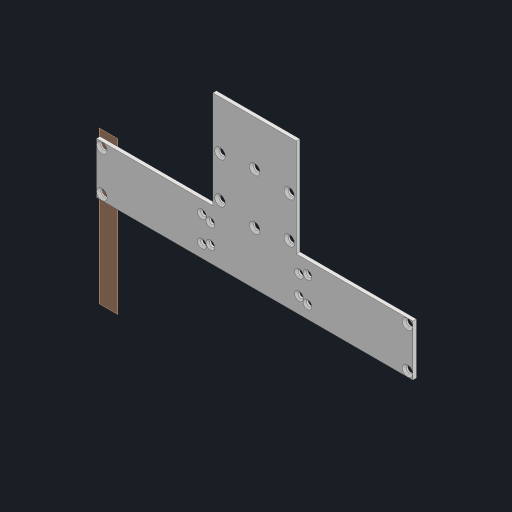
# Autodesk Inventor part: ceil
Saved by Autodesk Inventor 2023 (Build 270158000, 158)
## iProperties
Created: 2024-04-25
Part Number: ceil
Material: Generic
Document SubType Name: Modeling
Designer: szymo
Density: 1 g/cm^3
Appearance: Default
Author: szymo
Autodesk Inventor part; units mm, degrees
ref_plane "YZ Plane" through (0, 0, 0) normal (1, 0, 0) x (0, 1, 0)
ref_plane "XZ Plane" through (0, 0, 0) normal (0, 1, 0) x (-1, 0, 0)
ref_plane "XY Plane" through (0, 0, 0) normal (0, 0, 1) x (1, 0, 0)
ref_plane "Work Plane1" through (0, 0, 0) normal (0, 0, 1) x (1, 0, 0)
ref_plane "Work Plane2" through (0, 0, 0) normal (0, 0, 1) x (1, 0, 0)
sketch "Sketch3" plane through (0, 0, 0) normal (0, 0, 1) x (1, 0, 0)
  circle A0 centre (3, -25.75) radius 2.3 projected
  circle A1 centre (3, -3) radius 2.3 projected
  circle A2 centre (3, -74.8889) radius 2.3 projected
  line L0 (0, 0) -> (6, 0) projected
  line L1 (0, -77.8889) -> (0, 0) projected
  line L2 (0, -77.8889) -> (6, -77.8889) projected
  line L3 (6, -71.8889) -> (6, -77.8889) projected
  line L4 (6, -71.8889) -> (1.6, -71.8889) projected
  line L5 (1.6, -71.8889) -> (1.6, -56.7889) projected
  line L6 (1.6, -56.7889) -> (9.6, -56.7889) projected
  line L7 (9.6, -44.7889) -> (9.6, -56.7889) projected
  line L8 (3, -44.7889) -> (9.6, -44.7889) projected
  line L9 (3, -28.75) -> (3, -44.7889) projected
  line L10 (3, -28.75) -> (6, -28.75) projected
  line L11 (6, -28.75) -> (6, -22.75) projected
  line L12 (6, -22.75) -> (3, -22.75) projected
  line L13 (3, -6) -> (3, -22.75) projected
  line L14 (3, -6) -> (6, -6) projected
  line L15 (6, -6) -> (6, 0) projected
  circle A3 centre (5.6, -52.7889) radius 2.6 projected
  circle A4 centre (175, -3) radius 2.3 projected
  circle A5 centre (175, -25.75) radius 2.3 projected
  line L16 (175, -28.75) -> (175, -41.8889) projected
  line L17 (168.4, -41.8889) -> (175, -41.8889) projected
  line L18 (168.4, -53.8889) -> (168.4, -41.8889) projected
  line L19 (175, -53.8889) -> (168.4, -53.8889) projected
  line L20 (175, -53.8889) -> (175, -71.8889) projected
  line L21 (175, -71.8889) -> (172, -71.8889) projected
  line L22 (172, -71.8889) -> (172, -77.8889) projected
  line L23 (178, -77.8889) -> (172, -77.8889) projected
  line L24 (178, -77.8889) -> (178, 0) projected
  line L25 (178, 0) -> (172, 0) projected
  line L26 (172, 0) -> (172, -6) projected
  line L27 (172, -6) -> (175, -6) projected
  line L28 (175, -6) -> (175, -22.75) projected
  line L29 (175, -22.75) -> (172, -22.75) projected
  line L30 (172, -22.75) -> (172, -28.75) projected
  line L31 (172, -28.75) -> (175, -28.75) projected
  circle A6 centre (175, -74.8889) radius 2.3 projected
  circle A7 centre (172.4, -49.8889) radius 2.6 projected
  circle A8 centre (89, 0.9661) radius 2.3 projected
  circle A9 centre (89, 29.5) radius 2.3 projected
  circle A10 centre (89, 15.55) radius 3.3 projected
  circle A11 centre (89, -14.375) radius 3.3 projected
  circle A12 centre (89, 41.2) radius 3.3 projected
  line L32 (93.5, -27.75) -> (84.5, -27.75) projected
  line L33 (93.5, 55) -> (93.5, -27.75) projected
  line L34 (84.5, 55) -> (93.5, 55) projected
  line L35 (84.5, -27.75) -> (84.5, 55) projected
  line L36 (105.5, -27.75) -> (111.5, -27.75) projected
  line L37 (111.5, -24.9105) -> (111.5, -27.75) projected
  arc A13 (105.5, -24.9105) -> (111.5, -24.9105) centre (108.5, -23.95) ccw projected
  line L38 (105.5, -27.75) -> (105.5, -24.9105) projected
  arc A14 (111.5, -22.9895) -> (105.5, -22.9895) centre (108.5, -23.95) ccw projected
  line L39 (111.5, -5.5855) -> (111.5, -22.9895) projected
  arc A15 (105.5, -5.5855) -> (111.5, -5.5855) centre (108.5, -4.625) ccw projected
  line L40 (105.5, -22.9895) -> (105.5, -5.5855) projected
  circle A16 centre (108.4846, 4.5875) radius 2.3 projected
  arc A17 (105.5, 12.8395) -> (111.5, 12.8395) centre (108.5, 13.8) ccw projected
  line L41 (105.5, -3.6645) -> (105.5, 12.8395) projected
  arc A18 (111.5, -3.6645) -> (105.5, -3.6645) centre (108.5, -4.625) ccw projected
  line L42 (111.5, 12.8395) -> (111.5, -3.6645) projected
  circle A19 centre (108.4462, 27.5) radius 2.3 projected
  arc A20 (111.5, 14.7605) -> (105.5, 14.7605) centre (108.5, 13.8) ccw projected
  line L43 (111.5, 40.6331) -> (111.5, 14.7605) projected
  arc A21 (105.5, 40.1338) -> (111.5, 40.6331) centre (108.4231, 41.3077) ccw projected
  line L44 (105.5, 14.7605) -> (105.5, 40.1338) projected
  arc A22 (111.5, 41.9823) -> (105.5, 42.4816) centre (108.4231, 41.3077) ccw projected
  line L45 (111.5, 55) -> (111.5, 41.9823) projected
  line L46 (105.5, 55) -> (111.5, 55) projected
  line L47 (105.5, 42.4816) -> (105.5, 55) projected
  line L48 (111.5, 41.9823) -> (111.5, 55) projected
  line L49 (111.5, 41.9823) -> (112.5, 41.9823) projected
  line L50 (112.5, 41.9823) -> (112.5, 55) projected
  line L51 (111.5, 55) -> (112.5, 55) projected
  line L52 (111.5, 14.7605) -> (111.5, 40.6331) projected
  line L53 (111.5, 14.7605) -> (112.5, 14.7605) projected
  line L54 (112.5, 14.7605) -> (112.5, 40.6331) projected
  line L55 (111.5, 40.6331) -> (112.5, 40.6331) projected
  line L56 (111.5, -3.6645) -> (111.5, 12.8395) projected
  line L57 (111.5, -3.6645) -> (112.5, -3.6645) projected
  line L58 (112.5, -3.6645) -> (112.5, 12.8395) projected
  line L59 (111.5, 12.8395) -> (112.5, 12.8395) projected
  line L60 (66.5, 14.7605) -> (66.5, 40.6331) projected
  line L61 (66.5, 40.6331) -> (65.5, 40.6331) projected
  line L62 (65.5, 14.7605) -> (65.5, 40.6331) projected
  line L63 (66.5, 14.7605) -> (65.5, 14.7605) projected
  line L64 (66.5, 41.9823) -> (66.5, 55) projected
  line L65 (66.5, 55) -> (65.5, 55) projected
  line L66 (65.5, 41.9823) -> (65.5, 55) projected
  line L67 (66.5, 41.9823) -> (65.5, 41.9823) projected
  line L68 (66.5, -3.6645) -> (66.5, 12.8395) projected
  line L69 (66.5, 12.8395) -> (65.5, 12.8395) projected
  line L70 (65.5, -3.6645) -> (65.5, 12.8395) projected
  line L71 (66.5, -3.6645) -> (65.5, -3.6645) projected
  arc A23 (66.5, -5.5855) -> (72.5, -5.5855) centre (69.5, -4.625) ccw projected
  line L72 (66.5, -22.9895) -> (66.5, -5.5855) projected
  arc A24 (72.5, -22.9895) -> (66.5, -22.9895) centre (69.5, -23.95) ccw projected
  line L73 (72.5, -5.5855) -> (72.5, -22.9895) projected
  line L74 (66.5, -27.75) -> (72.5, -27.75) projected
  line L75 (72.5, -24.9105) -> (72.5, -27.75) projected
  arc A25 (66.5, -24.9105) -> (72.5, -24.9105) centre (69.5, -23.95) ccw projected
  line L76 (66.5, -27.75) -> (66.5, -24.9105) projected
  circle A26 centre (69.5, 4.5875) radius 2.3 projected
  arc A27 (72.5, -3.6645) -> (66.5, -3.6645) centre (69.5, -4.625) ccw projected
  line L77 (72.5, 12.8395) -> (72.5, -3.6645) projected
  arc A28 (66.5, 12.8395) -> (72.5, 12.8395) centre (69.5, 13.8) ccw projected
  line L78 (66.5, -3.6645) -> (66.5, 12.8395) projected
  circle A29 centre (69.5, 27.5) radius 2.3 projected
  arc A30 (66.5, 40.6331) -> (72.5, 40.1338) centre (69.5769, 41.3077) ccw projected
  line L79 (66.5, 14.7605) -> (66.5, 40.6331) projected
  arc A31 (72.5, 14.7605) -> (66.5, 14.7605) centre (69.5, 13.8) ccw projected
  line L80 (72.5, 40.1338) -> (72.5, 14.7605) projected
  arc A32 (72.5, 42.4816) -> (66.5, 41.9823) centre (69.5769, 41.3077) ccw projected
  line L81 (72.5, 55) -> (72.5, 42.4816) projected
  line L82 (66.5, 55) -> (72.5, 55) projected
  line L83 (66.5, 41.9823) -> (66.5, 55) projected
  circle A33 centre (59.3, -21.5445) radius 1.75 projected
  circle A34 centre (59.3, -7.2055) radius 1.75 projected
  line L84 (56.8, -28.75) -> (56.8, 0) projected
  line L85 (61.8, -28.75) -> (56.8, -28.75) projected
  line L86 (61.8, 0) -> (61.8, -28.75) projected
  line L87 (61.8, 0) -> (56.8, 0) projected
  circle A35 centre (64.05, -19.8657) radius 1.75 projected
  circle A36 centre (64.05, -8.8843) radius 1.75 projected
  line L88 (61.8, 0) -> (61.8, -28.75) projected
  line L89 (61.8, -28.75) -> (66.3, -28.75) projected
  line L90 (66.3, 0) -> (66.3, -28.75) projected
  line L91 (61.8, 0) -> (66.3, 0) projected
  circle A37 centre (113.95, -19.8657) radius 1.75 projected
  circle A38 centre (113.95, -8.8843) radius 1.75 projected
  line L92 (116.2, 0) -> (116.2, -28.75) projected
  line L93 (116.2, 0) -> (111.7, 0) projected
  line L94 (111.7, 0) -> (111.7, -28.75) projected
  line L95 (116.2, -28.75) -> (111.7, -28.75) projected
  circle A39 centre (118.7, -21.5445) radius 1.75 projected
  circle A40 centre (118.7, -7.2055) radius 1.75 projected
  line L96 (121.2, -28.75) -> (121.2, 0) projected
  line L97 (116.2, 0) -> (121.2, 0) projected
  line L98 (116.2, 0) -> (116.2, -28.75) projected
  line L99 (116.2, -28.75) -> (121.2, -28.75) projected
  line L100 (0, 0) -> (178, 0)
  line L101 (178, 0) -> (178, -28.75)
  line L102 (178, -28.75) -> (0, -28.75)
  line L103 (0, -28.75) -> (0, 0)
  line L104 (112.5, 0) -> (65.5, 0)
  line L105 (65.5, 0) -> (65.5, 55)
  line L106 (65.5, 55) -> (112.5, 55)
  line L107 (112.5, 55) -> (112.5, 0)
  point P0 (112.5, 0)
  point P1 (65.5, 0)
  point P2 (0, -28.75)
  point P3 (172, 0)
  constraints: 16 end point, 4 parallel, 3 point on line, 2 horizontal, 2 perpendicular
extrude "Extrusion2" add sketch "Sketch3" along normal blind 2 contours A0 | A1 | L0 L15 L14 L13 L12 L11 L10 L102 L1 | L100 L84 L102 L11 L12 L13 L14 L15 | L87 L86 L85 L84 | L91 L70 L71 L90 L89 L86 | L91 L90 L71 L70 | L70 L69 L68 L100 L91 | L90 L71 A27 L77 L100 L35 L32 L33 L41 A18 L57 L94 L102 | L105 L63 A31 L80 A30 L61 L67 A32 L81 L106 L35 L100 L77 A28 L69 | L100 L68 L71 L90 | L94 L57 L58 L93 L92 L95 | A28 L77 L100 L68 | L62 L61 L60 L63 | L100 L77 A27 L68 | L94 L93 L58 L57 | L57 L42 L100 L94 | L92 L97 L96 L99 | L60 A30 L80 A31 | A18 L41 L100 L42 | L100 L42 L59 L58 L93 | L96 L100 L26 L27 L28 L29 L30 L102 | L66 L65 L64 L67 | L100 A8 L33 L32 L35 | L35 L34 L33 L100 A8 | L100 L41 A17 L42 | L30 L29 L28 L27 L26 L25 L24 L102 L31 | L64 L82 L81 A32 | L100 A8 | A8 L100 | L100 L33 L106 L47 A22 L49 L107 L55 A21 L44 A20 L53 L59 A17 L41 | L53 L43 L55 L54 | L46 L45 A22 L47 | A20 L44 A21 L43 | L51 L50 L49 L45 | A4 | A5 | A9 | A10 | A11 | A12 | L38 A13 L37 L36 | A14 L40 A15 L39 | A16 | A19 | A23 L73 A24 L72 | L76 A25 L75 L74 | A26 | A29 | A33 | A34 | A35 | A36 | A37 | A38 | A39 | A40
sketch "Sketch4" plane through (0, 0, 2) normal (0, 0, 1) x (1, 0, 0)
  circle A0 centre (69.5, 27.5) radius 2.3 projected
  circle A1 centre (69.5, 4.5875) radius 2.3 projected
  circle A2 centre (89, 0.9661) radius 2 projected
  circle A3 centre (89, 29.5) radius 2.3 projected
  circle A4 centre (108.4462, 27.5) radius 2.3 projected
  circle A5 centre (108.4846, 4.5875) radius 2.3 projected
  circle A6 centre (64.05, -8.8843) radius 1.75 projected
  circle A7 centre (59.3, -7.2055) radius 1.75 projected
  circle A8 centre (59.3, -21.5445) radius 1.75 projected
  circle A9 centre (64.05, -19.8657) radius 1.75 projected
  circle A10 centre (118.7, -21.5445) radius 1.75 projected
  circle A11 centre (113.95, -19.8657) radius 1.75 projected
  circle A12 centre (113.95, -8.8843) radius 1.75 projected
  circle A13 centre (118.7, -7.2055) radius 1.75 projected
  circle A14 centre (3, -25.75) radius 2.3 projected
  circle A15 centre (3, -3) radius 2.3 projected
  circle A16 centre (175, -25.75) radius 2.3 projected
  circle A17 centre (175, -3) radius 2.3 projected
  point P0 (0, 0)
  constraints: 18 coincident
hole "Hole2" at (3, -3, 2) at (3, -25.75, 2) at (175, -3, 2) at (175, -25.75, 2) at (108.4846, 4.5875, 2) at (89, 0.9661, 2) at (69.5, 4.5875, 2) at (69.5, 27.5, 2) at (89, 29.5, 2) at (108.4462, 27.5, 2) direction (0, 0, -1) diameter 3.6 end through all countersink diameter 6 countersink angle 90 clearance for "Countersunk Flat Head Screw ISO 2009/7046" size "M3" standard "ISO"
sketch "Sketch5" plane through (0, 0, 2) normal (0, 0, 1) x (1, 0, 0)
  circle A0 centre (64.05, -19.8657) radius 1.75 projected
  circle A1 centre (59.3, -21.5445) radius 1.75 projected
  circle A2 centre (59.3, -7.2055) radius 1.75 projected
  circle A3 centre (64.05, -8.8843) radius 1.75 projected
  circle A4 centre (113.95, -8.8843) radius 1.75 projected
  circle A5 centre (118.7, -7.2055) radius 1.75 projected
  circle A6 centre (118.7, -21.5445) radius 1.75 projected
  circle A7 centre (113.95, -19.8657) radius 1.75 projected
  point P0 (0, 0)
  constraints: 8 coincident
hole "Hole3" at (59.3, -7.2055, 2) at (64.05, -8.8843, 2) at (64.05, -19.8657, 2) at (59.3, -21.5445, 2) at (113.95, -8.8843, 2) at (118.7, -7.2055, 2) at (118.7, -21.5445, 2) at (113.95, -19.8657, 2) direction (0, 0, -1) diameter 3.1 end through all countersink diameter 5 countersink angle 90 clearance for "Countersunk Flat Head Screw ISO 2009/7046" size "M2.5" standard "ISO"
body "Solid2"
